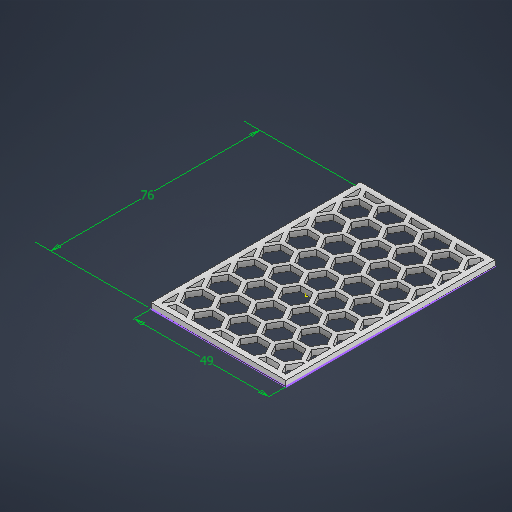
# Autodesk Inventor part: honneypattern
Saved by Autodesk Inventor 2026.1 (Build 301233020, 233B)
## iProperties
Created: 2026-01-08
Part Number: honneypattern
Material: Generic
Document SubType Name: Modeling
Designer: Paweł
Density: 1 g/cm^3
Appearance: Default
Author: Paweł
Autodesk Inventor part; units mm, degrees
ref_plane "YZ Plane" through (0, 0, 0) normal (1, 0, 0) x (0, 1, 0)
ref_plane "XZ Plane" through (0, 0, 0) normal (0, 1, 0) x (-1, 0, 0)
ref_plane "XY Plane" through (0, 0, 0) normal (0, 0, 1) x (1, 0, 0)
sketch "Sketch1" plane through (0, 0, 0) normal (0, 1, 0) x (-1, 0, 0)
  line L0 (23.9507, 32.8498) -> (-25.0493, 32.8498)
  line L1 (-25.0493, 32.8498) -> (-25.0493, -43.1502)
  line L2 (-25.0493, -43.1502) -> (23.9507, -43.1502)
  line L3 (23.9507, -43.1502) -> (23.9507, 32.8498)
  point P0 (0, 0)
  dimension "d0" = 49
  dimension "d1" = 76
  constraints: 8 end point, 2 parallel, 1 horizontal, 1 perpendicular
  measures "d0" distance of L0.start L0.end
  measures "d1" distance of L2.end L0.start
extrude "Extrusion1" add sketch "Sketch1" along normal blind 2
sketch "Sketch2" plane through (0, 2, 0) normal (0, 1, 0) x (1, 0, 0)
  line L0 (2.3094, -38.3498) -> (4.6188, -42.3498)
  line L1 (4.6188, -42.3498) -> (2.3094, -46.3498)
  line L2 (2.3094, -46.3498) -> (-2.3094, -46.3498)
  line L3 (-2.3094, -46.3498) -> (-4.6188, -42.3498)
  line L4 (-4.6188, -42.3498) -> (-2.3094, -38.3498)
  line L5 (-2.3094, -38.3498) -> (2.3094, -38.3498)
  line L6 (-23.9507, -32.8498) -> (25.0493, -32.8498) construction
  line L7 (-23.9507, 43.1502) -> (-23.9507, -32.8498) construction
  line L8 (-23.9507, -32.8498) -> (-23.9507, 0) construction
  line L9 (2.3094, -28.8498) -> (4.6188, -32.8498)
  line L10 (4.6188, -32.8498) -> (2.3094, -36.8498)
  line L11 (2.3094, -36.8498) -> (-2.3094, -36.8498)
  line L12 (-2.3094, -36.8498) -> (-4.6188, -32.8498)
  line L13 (-4.6188, -32.8498) -> (-2.3094, -28.8498)
  line L14 (-2.3094, -28.8498) -> (2.3094, -28.8498)
  line L15 (2.3094, -19.3498) -> (4.6188, -23.3498)
  line L16 (4.6188, -23.3498) -> (2.3094, -27.3498)
  line L17 (2.3094, -27.3498) -> (-2.3094, -27.3498)
  line L18 (-2.3094, -27.3498) -> (-4.6188, -23.3498)
  line L19 (-4.6188, -23.3498) -> (-2.3094, -19.3498)
  line L20 (-2.3094, -19.3498) -> (2.3094, -19.3498)
  line L21 (2.3094, -9.8498) -> (4.6188, -13.8498)
  line L22 (4.6188, -13.8498) -> (2.3094, -17.8498)
  line L23 (2.3094, -17.8498) -> (-2.3094, -17.8498)
  line L24 (-2.3094, -17.8498) -> (-4.6188, -13.8498)
  line L25 (-4.6188, -13.8498) -> (-2.3094, -9.8498)
  line L26 (-2.3094, -9.8498) -> (2.3094, -9.8498)
  line L27 (2.3094, -0.3498) -> (4.6188, -4.3498)
  line L28 (4.6188, -4.3498) -> (2.3094, -8.3498)
  line L29 (2.3094, -8.3498) -> (-2.3094, -8.3498)
  line L30 (-2.3094, -8.3498) -> (-4.6188, -4.3498)
  line L31 (-4.6188, -4.3498) -> (-2.3094, -0.3498)
  line L32 (-2.3094, -0.3498) -> (2.3094, -0.3498)
  line L33 (2.3094, 9.1502) -> (4.6188, 5.1502)
  line L34 (4.6188, 5.1502) -> (2.3094, 1.1502)
  line L35 (2.3094, 1.1502) -> (-2.3094, 1.1502)
  line L36 (-2.3094, 1.1502) -> (-4.6188, 5.1502)
  line L37 (-4.6188, 5.1502) -> (-2.3094, 9.1502)
  line L38 (-2.3094, 9.1502) -> (2.3094, 9.1502)
  line L39 (2.3094, 18.6502) -> (4.6188, 14.6502)
  line L40 (4.6188, 14.6502) -> (2.3094, 10.6502)
  line L41 (2.3094, 10.6502) -> (-2.3094, 10.6502)
  line L42 (-2.3094, 10.6502) -> (-4.6188, 14.6502)
  line L43 (-4.6188, 14.6502) -> (-2.3094, 18.6502)
  line L44 (-2.3094, 18.6502) -> (2.3094, 18.6502)
  line L45 (2.3094, 28.1502) -> (4.6188, 24.1502)
  line L46 (4.6188, 24.1502) -> (2.3094, 20.1502)
  line L47 (2.3094, 20.1502) -> (-2.3094, 20.1502)
  line L48 (-2.3094, 20.1502) -> (-4.6188, 24.1502)
  line L49 (-4.6188, 24.1502) -> (-2.3094, 28.1502)
  line L50 (-2.3094, 28.1502) -> (2.3094, 28.1502)
  line L51 (2.3094, 37.6502) -> (4.6188, 33.6502)
  line L52 (4.6188, 33.6502) -> (2.3094, 29.6502)
  line L53 (2.3094, 29.6502) -> (-2.3094, 29.6502)
  line L54 (-2.3094, 29.6502) -> (-4.6188, 33.6502)
  line L55 (-4.6188, 33.6502) -> (-2.3094, 37.6502)
  line L56 (-2.3094, 37.6502) -> (2.3094, 37.6502)
  line L57 (2.3094, 47.1502) -> (4.6188, 43.1502)
  line L58 (4.6188, 43.1502) -> (2.3094, 39.1502)
  line L59 (2.3094, 39.1502) -> (-2.3094, 39.1502)
  line L60 (-2.3094, 39.1502) -> (-4.6188, 43.1502)
  line L61 (-4.6188, 43.1502) -> (-2.3094, 47.1502)
  line L62 (-2.3094, 47.1502) -> (2.3094, 47.1502)
  line L63 (0, -42.3498) -> (-3.4641, -40.3498) construction
  line L64 (-10.5366, -14.5998) -> (-5.9178, -14.5998)
  line L65 (-5.9178, -13.0998) -> (-10.5366, -13.0998)
  line L66 (-10.5366, -13.0998) -> (-12.846, -9.0998)
  line L67 (-3.6084, -9.0998) -> (-5.9178, -13.0998)
  line L68 (-5.9178, -5.0998) -> (-3.6084, -9.0998)
  line L69 (-10.5366, -5.0998) -> (-5.9178, -5.0998)
  line L70 (-12.846, -9.0998) -> (-10.5366, -5.0998)
  line L71 (-5.9178, -3.5998) -> (-10.5366, -3.5998)
  line L72 (-5.9178, -24.0998) -> (-3.6084, -28.0998)
  line L73 (-12.846, -28.0998) -> (-10.5366, -24.0998)
  line L74 (-5.9178, -14.5998) -> (-3.6084, -18.5998)
  line L75 (-12.846, -18.5998) -> (-10.5366, -14.5998)
  line L76 (-3.6084, -18.5998) -> (-5.9178, -22.5998)
  line L77 (-10.5366, -22.5998) -> (-12.846, -18.5998)
  line L78 (-5.9178, -22.5998) -> (-10.5366, -22.5998)
  line L79 (-10.5366, -24.0998) -> (-5.9178, -24.0998)
  line L80 (-10.5366, -3.5998) -> (-12.846, 0.4002)
  line L81 (-3.6084, 0.4002) -> (-5.9178, -3.5998)
  line L82 (-12.846, 0.4002) -> (-10.5366, 4.4002)
  line L83 (-5.9178, 4.4002) -> (-3.6084, 0.4002)
  line L84 (-10.5366, 4.4002) -> (-5.9178, 4.4002)
  line L85 (-5.9178, 5.9002) -> (-10.5366, 5.9002)
  line L86 (-10.5366, 5.9002) -> (-12.846, 9.9002)
  line L87 (-3.6084, 9.9002) -> (-5.9178, 5.9002)
  line L88 (-12.846, 9.9002) -> (-10.5366, 13.9002)
  line L89 (-5.9178, 13.9002) -> (-3.6084, 9.9002)
  line L90 (-10.5366, 13.9002) -> (-5.9178, 13.9002)
  line L91 (-5.9178, 15.4002) -> (-10.5366, 15.4002)
  line L92 (-10.5366, 15.4002) -> (-12.846, 19.4002)
  line L93 (-3.6084, 19.4002) -> (-5.9178, 15.4002)
  line L94 (-5.9178, -33.5998) -> (-3.6084, -37.5998)
  line L95 (-3.6084, -37.5998) -> (-5.9178, -41.5998)
  line L96 (-5.9178, -41.5998) -> (-10.5366, -41.5998)
  line L97 (-10.5366, -41.5998) -> (-12.846, -37.5998)
  line L98 (-12.846, -37.5998) -> (-10.5366, -33.5998)
  line L99 (-10.5366, -33.5998) -> (-5.9178, -33.5998)
  line L100 (-3.6084, -28.0998) -> (-5.9178, -32.0998)
  line L101 (-5.9178, -32.0998) -> (-10.5366, -32.0998)
  line L102 (-10.5366, -32.0998) -> (-12.846, -28.0998)
  line L103 (-8.2272, -37.5998) -> (-11.6913, -35.5998) construction
  line L104 (-12.846, 19.4002) -> (-10.5366, 23.4002)
  line L105 (-5.9178, 23.4002) -> (-3.6084, 19.4002)
  line L106 (-10.5366, 23.4002) -> (-5.9178, 23.4002)
  line L107 (-5.9178, 24.9002) -> (-10.5366, 24.9002)
  line L108 (-10.5366, 24.9002) -> (-12.846, 28.9002)
  line L109 (-3.6084, 28.9002) -> (-5.9178, 24.9002)
  line L110 (-12.846, 28.9002) -> (-10.5366, 32.9002)
  line L111 (-5.9178, 32.9002) -> (-3.6084, 28.9002)
  line L112 (-5.9178, 34.4002) -> (-10.5366, 34.4002)
  line L113 (-3.6084, 38.4002) -> (-5.9178, 34.4002)
  line L114 (-10.5366, 34.4002) -> (-12.846, 38.4002)
  line L115 (-5.9178, 42.4002) -> (-3.6084, 38.4002)
  line L116 (-10.5366, 42.4002) -> (-5.9178, 42.4002)
  line L117 (-12.846, 38.4002) -> (-10.5366, 42.4002)
  line L118 (-10.5366, 32.9002) -> (-5.9178, 32.9002)
  line L119 (-10.5366, 43.9002) -> (-12.846, 47.9002)
  line L120 (-3.6084, 47.9002) -> (-5.9178, 43.9002)
  line L121 (-12.846, 47.9002) -> (-10.5366, 51.9002)
  line L122 (-10.5366, 51.9002) -> (-5.9178, 51.9002)
  line L123 (-5.9178, 51.9002) -> (-3.6084, 47.9002)
  line L124 (-5.9178, 43.9002) -> (-10.5366, 43.9002)
  line L125 (-18.7639, -9.8498) -> (-14.1451, -9.8498)
  line L126 (-14.1451, -8.3498) -> (-18.7639, -8.3498)
  line L127 (-18.7639, -8.3498) -> (-21.0733, -4.3498)
  line L128 (-11.8357, -4.3498) -> (-14.1451, -8.3498)
  line L129 (-14.1451, -0.3498) -> (-11.8357, -4.3498)
  line L130 (-18.7639, -0.3498) -> (-14.1451, -0.3498)
  line L131 (-21.0733, -4.3498) -> (-18.7639, -0.3498)
  line L132 (-14.1451, 1.1502) -> (-18.7639, 1.1502)
  line L133 (-14.1451, -19.3498) -> (-11.8357, -23.3498)
  line L134 (-21.0733, -23.3498) -> (-18.7639, -19.3498)
  line L135 (-14.1451, -9.8498) -> (-11.8357, -13.8498)
  line L136 (-21.0733, -13.8498) -> (-18.7639, -9.8498)
  line L137 (-11.8357, -13.8498) -> (-14.1451, -17.8498)
  line L138 (-18.7639, -17.8498) -> (-21.0733, -13.8498)
  line L139 (-14.1451, -17.8498) -> (-18.7639, -17.8498)
  line L140 (-18.7639, -19.3498) -> (-14.1451, -19.3498)
  line L141 (-18.7639, 1.1502) -> (-21.0733, 5.1502)
  line L142 (-11.8357, 5.1502) -> (-14.1451, 1.1502)
  line L143 (-21.0733, 5.1502) -> (-18.7639, 9.1502)
  line L144 (-14.1451, 9.1502) -> (-11.8357, 5.1502)
  line L145 (-18.7639, 9.1502) -> (-14.1451, 9.1502)
  line L146 (-14.1451, 10.6502) -> (-18.7639, 10.6502)
  line L147 (-18.7639, 10.6502) -> (-21.0733, 14.6502)
  line L148 (-11.8357, 14.6502) -> (-14.1451, 10.6502)
  line L149 (-21.0733, 14.6502) -> (-18.7639, 18.6502)
  line L150 (-14.1451, 18.6502) -> (-11.8357, 14.6502)
  line L151 (-18.7639, 18.6502) -> (-14.1451, 18.6502)
  line L152 (-14.1451, 20.1502) -> (-18.7639, 20.1502)
  line L153 (-18.7639, 20.1502) -> (-21.0733, 24.1502)
  line L154 (-11.8357, 24.1502) -> (-14.1451, 20.1502)
  line L155 (-14.1451, -28.8498) -> (-11.8357, -32.8498)
  line L156 (-11.8357, -32.8498) -> (-14.1451, -36.8498)
  line L157 (-14.1451, -36.8498) -> (-18.7639, -36.8498)
  line L158 (-18.7639, -36.8498) -> (-21.0733, -32.8498)
  line L159 (-21.0733, -32.8498) -> (-18.7639, -28.8498)
  line L160 (-18.7639, -28.8498) -> (-14.1451, -28.8498)
  line L161 (-11.8357, -23.3498) -> (-14.1451, -27.3498)
  line L162 (-14.1451, -27.3498) -> (-18.7639, -27.3498)
  line L163 (-18.7639, -27.3498) -> (-21.0733, -23.3498)
  line L164 (-16.4545, -32.8498) -> (-19.9186, -30.8498) construction
  line L165 (-21.0733, 24.1502) -> (-18.7639, 28.1502)
  line L166 (-14.1451, 28.1502) -> (-11.8357, 24.1502)
  line L167 (-18.7639, 28.1502) -> (-14.1451, 28.1502)
  line L168 (-14.1451, 29.6502) -> (-18.7639, 29.6502)
  line L169 (-18.7639, 29.6502) -> (-21.0733, 33.6502)
  line L170 (-11.8357, 33.6502) -> (-14.1451, 29.6502)
  line L171 (-21.0733, 33.6502) -> (-18.7639, 37.6502)
  line L172 (-14.1451, 37.6502) -> (-11.8357, 33.6502)
  line L173 (-14.1451, 39.1502) -> (-18.7639, 39.1502)
  line L174 (-11.8357, 43.1502) -> (-14.1451, 39.1502)
  line L175 (-18.7639, 39.1502) -> (-21.0733, 43.1502)
  line L176 (-14.1451, 47.1502) -> (-11.8357, 43.1502)
  line L177 (-18.7639, 47.1502) -> (-14.1451, 47.1502)
  line L178 (-21.0733, 43.1502) -> (-18.7639, 47.1502)
  line L179 (-18.7639, 37.6502) -> (-14.1451, 37.6502)
  line L180 (-18.7639, 48.6502) -> (-21.0733, 52.6502)
  line L181 (-11.8357, 52.6502) -> (-14.1451, 48.6502)
  line L182 (-21.0733, 52.6502) -> (-18.7639, 56.6502)
  line L183 (-18.7639, 56.6502) -> (-14.1451, 56.6502)
  line L184 (-14.1451, 56.6502) -> (-11.8357, 52.6502)
  line L185 (-14.1451, 48.6502) -> (-18.7639, 48.6502)
  line L186 (-26.9911, -5.0998) -> (-22.3723, -5.0998)
  line L187 (-22.3723, -3.5998) -> (-26.9911, -3.5998)
  line L188 (-26.9911, -3.5998) -> (-29.3005, 0.4002)
  line L189 (-20.0629, 0.4002) -> (-22.3723, -3.5998)
  line L190 (-22.3723, 4.4002) -> (-20.0629, 0.4002)
  line L191 (-26.9911, 4.4002) -> (-22.3723, 4.4002)
  line L192 (-29.3005, 0.4002) -> (-26.9911, 4.4002)
  line L193 (-22.3723, 5.9002) -> (-26.9911, 5.9002)
  line L194 (-22.3723, -14.5998) -> (-20.0629, -18.5998)
  line L195 (-29.3005, -18.5998) -> (-26.9911, -14.5998)
  line L196 (-22.3723, -5.0998) -> (-20.0629, -9.0998)
  line L197 (-29.3005, -9.0998) -> (-26.9911, -5.0998)
  line L198 (-20.0629, -9.0998) -> (-22.3723, -13.0998)
  line L199 (-26.9911, -13.0998) -> (-29.3005, -9.0998)
  line L200 (-22.3723, -13.0998) -> (-26.9911, -13.0998)
  line L201 (-26.9911, -14.5998) -> (-22.3723, -14.5998)
  line L202 (-26.9911, 5.9002) -> (-29.3005, 9.9002)
  line L203 (-20.0629, 9.9002) -> (-22.3723, 5.9002)
  line L204 (-29.3005, 9.9002) -> (-26.9911, 13.9002)
  line L205 (-22.3723, 13.9002) -> (-20.0629, 9.9002)
  line L206 (-26.9911, 13.9002) -> (-22.3723, 13.9002)
  line L207 (-22.3723, 15.4002) -> (-26.9911, 15.4002)
  line L208 (-26.9911, 15.4002) -> (-29.3005, 19.4002)
  line L209 (-20.0629, 19.4002) -> (-22.3723, 15.4002)
  line L210 (-29.3005, 19.4002) -> (-26.9911, 23.4002)
  line L211 (-22.3723, 23.4002) -> (-20.0629, 19.4002)
  line L212 (-26.9911, 23.4002) -> (-22.3723, 23.4002)
  line L213 (-22.3723, 24.9002) -> (-26.9911, 24.9002)
  line L214 (-26.9911, 24.9002) -> (-29.3005, 28.9002)
  line L215 (-20.0629, 28.9002) -> (-22.3723, 24.9002)
  line L216 (-22.3723, -24.0998) -> (-20.0629, -28.0998)
  line L217 (-20.0629, -28.0998) -> (-22.3723, -32.0998)
  line L218 (-22.3723, -32.0998) -> (-26.9911, -32.0998)
  line L219 (-26.9911, -32.0998) -> (-29.3005, -28.0998)
  line L220 (-29.3005, -28.0998) -> (-26.9911, -24.0998)
  line L221 (-26.9911, -24.0998) -> (-22.3723, -24.0998)
  line L222 (-20.0629, -18.5998) -> (-22.3723, -22.5998)
  line L223 (-22.3723, -22.5998) -> (-26.9911, -22.5998)
  line L224 (-26.9911, -22.5998) -> (-29.3005, -18.5998)
  line L225 (-24.6817, -28.0998) -> (-28.1458, -26.0998) construction
  line L226 (-29.3005, 28.9002) -> (-26.9911, 32.9002)
  line L227 (-22.3723, 32.9002) -> (-20.0629, 28.9002)
  line L228 (-26.9911, 32.9002) -> (-22.3723, 32.9002)
  line L229 (-22.3723, 34.4002) -> (-26.9911, 34.4002)
  line L230 (-26.9911, 34.4002) -> (-29.3005, 38.4002)
  line L231 (-20.0629, 38.4002) -> (-22.3723, 34.4002)
  line L232 (-29.3005, 38.4002) -> (-26.9911, 42.4002)
  line L233 (-22.3723, 42.4002) -> (-20.0629, 38.4002)
  line L234 (-22.3723, 43.9002) -> (-26.9911, 43.9002)
  line L235 (-20.0629, 47.9002) -> (-22.3723, 43.9002)
  line L236 (-26.9911, 43.9002) -> (-29.3005, 47.9002)
  line L237 (-22.3723, 51.9002) -> (-20.0629, 47.9002)
  line L238 (-26.9911, 51.9002) -> (-22.3723, 51.9002)
  line L239 (-29.3005, 47.9002) -> (-26.9911, 51.9002)
  line L240 (-26.9911, 42.4002) -> (-22.3723, 42.4002)
  line L241 (-26.9911, 53.4002) -> (-29.3005, 57.4002)
  line L242 (-20.0629, 57.4002) -> (-22.3723, 53.4002)
  line L243 (-29.3005, 57.4002) -> (-26.9911, 61.4002)
  line L244 (-26.9911, 61.4002) -> (-22.3723, 61.4002)
  line L245 (-22.3723, 61.4002) -> (-20.0629, 57.4002)
  line L246 (-22.3723, 53.4002) -> (-26.9911, 53.4002)
  line L247 (10.5366, -43.0998) -> (12.846, -47.0998)
  line L248 (12.846, -47.0998) -> (10.5366, -51.0998)
  line L249 (10.5366, -51.0998) -> (5.9178, -51.0998)
  line L250 (5.9178, -51.0998) -> (3.6084, -47.0998)
  line L251 (3.6084, -47.0998) -> (5.9178, -43.0998)
  line L252 (8.2272, -47.0998) -> (4.7631, -45.0998) construction
  line L253 (12.846, -37.5998) -> (10.5366, -41.5998)
  line L254 (10.5366, -24.0998) -> (12.846, -28.0998)
  line L255 (12.846, -28.0998) -> (10.5366, -32.0998)
  line L256 (5.9178, -32.0998) -> (3.6084, -28.0998)
  line L257 (3.6084, -28.0998) -> (5.9178, -24.0998)
  line L258 (5.9178, -22.5998) -> (3.6084, -18.5998)
  line L259 (5.9178, -24.0998) -> (10.5366, -24.0998)
  line L260 (12.846, -9.0998) -> (10.5366, -13.0998)
  line L261 (10.5366, -13.0998) -> (5.9178, -13.0998)
  line L262 (5.9178, -14.5998) -> (10.5366, -14.5998)
  line L263 (10.5366, -14.5998) -> (12.846, -18.5998)
  line L264 (12.846, -18.5998) -> (10.5366, -22.5998)
  line L265 (10.5366, -22.5998) -> (5.9178, -22.5998)
  line L266 (3.6084, -18.5998) -> (5.9178, -14.5998)
  line L267 (5.9178, -13.0998) -> (3.6084, -9.0998)
  line L268 (5.9178, -3.5998) -> (3.6084, 0.4002)
  line L269 (3.6084, -9.0998) -> (5.9178, -5.0998)
  line L270 (5.9178, -5.0998) -> (10.5366, -5.0998)
  line L271 (10.5366, -3.5998) -> (5.9178, -3.5998)
  line L272 (10.5366, -5.0998) -> (12.846, -9.0998)
  line L273 (12.846, 0.4002) -> (10.5366, -3.5998)
  line L274 (10.5366, 4.4002) -> (12.846, 0.4002)
  line L275 (3.6084, 0.4002) -> (5.9178, 4.4002)
  line L276 (5.9178, 4.4002) -> (10.5366, 4.4002)
  line L277 (5.9178, 5.9002) -> (3.6084, 9.9002)
  line L278 (3.6084, 9.9002) -> (5.9178, 13.9002)
  line L279 (12.846, 9.9002) -> (10.5366, 5.9002)
  line L280 (5.9178, 13.9002) -> (10.5366, 13.9002)
  line L281 (10.5366, 15.4002) -> (5.9178, 15.4002)
  line L282 (10.5366, 13.9002) -> (12.846, 9.9002)
  line L283 (12.846, 19.4002) -> (10.5366, 15.4002)
  line L284 (10.5366, 5.9002) -> (5.9178, 5.9002)
  line L285 (5.9178, 15.4002) -> (3.6084, 19.4002)
  line L286 (3.6084, 19.4002) -> (5.9178, 23.4002)
  line L287 (3.6084, 28.9002) -> (5.9178, 32.9002)
  line L288 (5.9178, 24.9002) -> (3.6084, 28.9002)
  line L289 (10.5366, 32.9002) -> (12.846, 28.9002)
  line L290 (10.5366, 24.9002) -> (5.9178, 24.9002)
  line L291 (5.9178, 23.4002) -> (10.5366, 23.4002)
  line L292 (12.846, 28.9002) -> (10.5366, 24.9002)
  line L293 (10.5366, 23.4002) -> (12.846, 19.4002)
  line L294 (5.9178, 32.9002) -> (10.5366, 32.9002)
  line L295 (3.6084, 38.4002) -> (5.9178, 42.4002)
  line L296 (5.9178, 42.4002) -> (10.5366, 42.4002)
  line L297 (10.5366, 34.4002) -> (5.9178, 34.4002)
  line L298 (10.5366, 42.4002) -> (12.846, 38.4002)
  line L299 (12.846, 38.4002) -> (10.5366, 34.4002)
  line L300 (5.9178, 34.4002) -> (3.6084, 38.4002)
  line L301 (10.5366, -41.5998) -> (5.9178, -41.5998)
  line L302 (5.9178, -43.0998) -> (10.5366, -43.0998)
  line L303 (10.5366, -33.5998) -> (12.846, -37.5998)
  line L304 (5.9178, -41.5998) -> (3.6084, -37.5998)
  line L305 (5.9178, -33.5998) -> (10.5366, -33.5998)
  line L306 (10.5366, -32.0998) -> (5.9178, -32.0998)
  line L307 (3.6084, -37.5998) -> (5.9178, -33.5998)
  line L308 (18.7639, -47.8498) -> (21.0733, -51.8498)
  line L309 (21.0733, -51.8498) -> (18.7639, -55.8498)
  line L310 (18.7639, -55.8498) -> (14.1451, -55.8498)
  line L311 (14.1451, -55.8498) -> (11.8357, -51.8498)
  line L312 (11.8357, -51.8498) -> (14.1451, -47.8498)
  line L313 (16.4545, -51.8498) -> (12.9904, -49.8498) construction
  line L314 (21.0733, -42.3498) -> (18.7639, -46.3498)
  line L315 (18.7639, -28.8498) -> (21.0733, -32.8498)
  line L316 (21.0733, -32.8498) -> (18.7639, -36.8498)
  line L317 (14.1451, -36.8498) -> (11.8357, -32.8498)
  line L318 (11.8357, -32.8498) -> (14.1451, -28.8498)
  line L319 (14.1451, -27.3498) -> (11.8357, -23.3498)
  line L320 (14.1451, -28.8498) -> (18.7639, -28.8498)
  line L321 (21.0733, -13.8498) -> (18.7639, -17.8498)
  line L322 (18.7639, -17.8498) -> (14.1451, -17.8498)
  line L323 (14.1451, -19.3498) -> (18.7639, -19.3498)
  line L324 (18.7639, -19.3498) -> (21.0733, -23.3498)
  line L325 (21.0733, -23.3498) -> (18.7639, -27.3498)
  line L326 (18.7639, -27.3498) -> (14.1451, -27.3498)
  line L327 (11.8357, -23.3498) -> (14.1451, -19.3498)
  line L328 (14.1451, -17.8498) -> (11.8357, -13.8498)
  line L329 (14.1451, -8.3498) -> (11.8357, -4.3498)
  line L330 (11.8357, -13.8498) -> (14.1451, -9.8498)
  line L331 (14.1451, -9.8498) -> (18.7639, -9.8498)
  line L332 (18.7639, -8.3498) -> (14.1451, -8.3498)
  line L333 (18.7639, -9.8498) -> (21.0733, -13.8498)
  line L334 (21.0733, -4.3498) -> (18.7639, -8.3498)
  line L335 (18.7639, -0.3498) -> (21.0733, -4.3498)
  line L336 (11.8357, -4.3498) -> (14.1451, -0.3498)
  line L337 (14.1451, -0.3498) -> (18.7639, -0.3498)
  line L338 (14.1451, 1.1502) -> (11.8357, 5.1502)
  line L339 (11.8357, 5.1502) -> (14.1451, 9.1502)
  line L340 (21.0733, 5.1502) -> (18.7639, 1.1502)
  line L341 (14.1451, 9.1502) -> (18.7639, 9.1502)
  line L342 (18.7639, 10.6502) -> (14.1451, 10.6502)
  line L343 (18.7639, 9.1502) -> (21.0733, 5.1502)
  line L344 (21.0733, 14.6502) -> (18.7639, 10.6502)
  line L345 (18.7639, 1.1502) -> (14.1451, 1.1502)
  line L346 (14.1451, 10.6502) -> (11.8357, 14.6502)
  line L347 (11.8357, 14.6502) -> (14.1451, 18.6502)
  line L348 (11.8357, 24.1502) -> (14.1451, 28.1502)
  line L349 (14.1451, 20.1502) -> (11.8357, 24.1502)
  line L350 (18.7639, 28.1502) -> (21.0733, 24.1502)
  line L351 (18.7639, 20.1502) -> (14.1451, 20.1502)
  line L352 (14.1451, 18.6502) -> (18.7639, 18.6502)
  line L353 (21.0733, 24.1502) -> (18.7639, 20.1502)
  line L354 (18.7639, 18.6502) -> (21.0733, 14.6502)
  line L355 (14.1451, 28.1502) -> (18.7639, 28.1502)
  line L356 (11.8357, 33.6502) -> (14.1451, 37.6502)
  line L357 (14.1451, 37.6502) -> (18.7639, 37.6502)
  line L358 (18.7639, 29.6502) -> (14.1451, 29.6502)
  line L359 (18.7639, 37.6502) -> (21.0733, 33.6502)
  line L360 (21.0733, 33.6502) -> (18.7639, 29.6502)
  line L361 (14.1451, 29.6502) -> (11.8357, 33.6502)
  line L362 (18.7639, -46.3498) -> (14.1451, -46.3498)
  line L363 (14.1451, -47.8498) -> (18.7639, -47.8498)
  line L364 (18.7639, -38.3498) -> (21.0733, -42.3498)
  line L365 (14.1451, -46.3498) -> (11.8357, -42.3498)
  line L366 (14.1451, -38.3498) -> (18.7639, -38.3498)
  line L367 (18.7639, -36.8498) -> (14.1451, -36.8498)
  line L368 (11.8357, -42.3498) -> (14.1451, -38.3498)
  line L369 (26.9911, -52.5998) -> (29.3005, -56.5998)
  line L370 (29.3005, -56.5998) -> (26.9911, -60.5998)
  line L371 (26.9911, -60.5998) -> (22.3723, -60.5998)
  line L372 (22.3723, -60.5998) -> (20.0629, -56.5998)
  line L373 (20.0629, -56.5998) -> (22.3723, -52.5998)
  line L374 (24.6817, -56.5998) -> (21.2176, -54.5998) construction
  line L375 (29.3005, -47.0998) -> (26.9911, -51.0998)
  line L376 (26.9911, -33.5998) -> (29.3005, -37.5998)
  line L377 (29.3005, -37.5998) -> (26.9911, -41.5998)
  line L378 (22.3723, -41.5998) -> (20.0629, -37.5998)
  line L379 (20.0629, -37.5998) -> (22.3723, -33.5998)
  line L380 (22.3723, -32.0998) -> (20.0629, -28.0998)
  line L381 (22.3723, -33.5998) -> (26.9911, -33.5998)
  line L382 (29.3005, -18.5998) -> (26.9911, -22.5998)
  line L383 (26.9911, -22.5998) -> (22.3723, -22.5998)
  line L384 (22.3723, -24.0998) -> (26.9911, -24.0998)
  line L385 (26.9911, -24.0998) -> (29.3005, -28.0998)
  line L386 (29.3005, -28.0998) -> (26.9911, -32.0998)
  line L387 (26.9911, -32.0998) -> (22.3723, -32.0998)
  line L388 (20.0629, -28.0998) -> (22.3723, -24.0998)
  line L389 (22.3723, -22.5998) -> (20.0629, -18.5998)
  line L390 (22.3723, -13.0998) -> (20.0629, -9.0998)
  line L391 (20.0629, -18.5998) -> (22.3723, -14.5998)
  line L392 (22.3723, -14.5998) -> (26.9911, -14.5998)
  line L393 (26.9911, -13.0998) -> (22.3723, -13.0998)
  line L394 (26.9911, -14.5998) -> (29.3005, -18.5998)
  line L395 (29.3005, -9.0998) -> (26.9911, -13.0998)
  line L396 (26.9911, -5.0998) -> (29.3005, -9.0998)
  line L397 (20.0629, -9.0998) -> (22.3723, -5.0998)
  line L398 (22.3723, -5.0998) -> (26.9911, -5.0998)
  line L399 (22.3723, -3.5998) -> (20.0629, 0.4002)
  line L400 (20.0629, 0.4002) -> (22.3723, 4.4002)
  line L401 (29.3005, 0.4002) -> (26.9911, -3.5998)
  line L402 (22.3723, 4.4002) -> (26.9911, 4.4002)
  line L403 (26.9911, 5.9002) -> (22.3723, 5.9002)
  line L404 (26.9911, 4.4002) -> (29.3005, 0.4002)
  line L405 (29.3005, 9.9002) -> (26.9911, 5.9002)
  line L406 (26.9911, -3.5998) -> (22.3723, -3.5998)
  line L407 (22.3723, 5.9002) -> (20.0629, 9.9002)
  line L408 (20.0629, 9.9002) -> (22.3723, 13.9002)
  line L409 (20.0629, 19.4002) -> (22.3723, 23.4002)
  line L410 (22.3723, 15.4002) -> (20.0629, 19.4002)
  line L411 (26.9911, 23.4002) -> (29.3005, 19.4002)
  line L412 (26.9911, 15.4002) -> (22.3723, 15.4002)
  line L413 (22.3723, 13.9002) -> (26.9911, 13.9002)
  line L414 (29.3005, 19.4002) -> (26.9911, 15.4002)
  line L415 (26.9911, 13.9002) -> (29.3005, 9.9002)
  line L416 (22.3723, 23.4002) -> (26.9911, 23.4002)
  line L417 (20.0629, 28.9002) -> (22.3723, 32.9002)
  line L418 (22.3723, 32.9002) -> (26.9911, 32.9002)
  line L419 (26.9911, 24.9002) -> (22.3723, 24.9002)
  line L420 (26.9911, 32.9002) -> (29.3005, 28.9002)
  line L421 (29.3005, 28.9002) -> (26.9911, 24.9002)
  line L422 (22.3723, 24.9002) -> (20.0629, 28.9002)
  line L423 (26.9911, -51.0998) -> (22.3723, -51.0998)
  line L424 (22.3723, -52.5998) -> (26.9911, -52.5998)
  line L425 (26.9911, -43.0998) -> (29.3005, -47.0998)
  line L426 (22.3723, -51.0998) -> (20.0629, -47.0998)
  line L427 (22.3723, -43.0998) -> (26.9911, -43.0998)
  line L428 (26.9911, -41.5998) -> (22.3723, -41.5998)
  line L429 (20.0629, -47.0998) -> (22.3723, -43.0998)
  line L430 (35.2184, -57.3498) -> (37.5278, -61.3498)
  line L431 (37.5278, -61.3498) -> (35.2184, -65.3498)
  line L432 (35.2184, -65.3498) -> (30.5996, -65.3498)
  line L433 (30.5996, -65.3498) -> (28.2902, -61.3498)
  line L434 (28.2902, -61.3498) -> (30.5996, -57.3498)
  line L435 (32.909, -61.3498) -> (29.4449, -59.3498) construction
  line L436 (37.5278, -51.8498) -> (35.2184, -55.8498)
  line L437 (35.2184, -38.3498) -> (37.5278, -42.3498)
  line L438 (37.5278, -42.3498) -> (35.2184, -46.3498)
  line L439 (30.5996, -46.3498) -> (28.2902, -42.3498)
  line L440 (28.2902, -42.3498) -> (30.5996, -38.3498)
  line L441 (30.5996, -36.8498) -> (28.2902, -32.8498)
  line L442 (30.5996, -38.3498) -> (35.2184, -38.3498)
  line L443 (37.5278, -23.3498) -> (35.2184, -27.3498)
  line L444 (35.2184, -27.3498) -> (30.5996, -27.3498)
  line L445 (30.5996, -28.8498) -> (35.2184, -28.8498)
  line L446 (35.2184, -28.8498) -> (37.5278, -32.8498)
  line L447 (37.5278, -32.8498) -> (35.2184, -36.8498)
  line L448 (35.2184, -36.8498) -> (30.5996, -36.8498)
  line L449 (28.2902, -32.8498) -> (30.5996, -28.8498)
  line L450 (30.5996, -27.3498) -> (28.2902, -23.3498)
  line L451 (30.5996, -17.8498) -> (28.2902, -13.8498)
  line L452 (28.2902, -23.3498) -> (30.5996, -19.3498)
  line L453 (30.5996, -19.3498) -> (35.2184, -19.3498)
  line L454 (35.2184, -17.8498) -> (30.5996, -17.8498)
  line L455 (35.2184, -19.3498) -> (37.5278, -23.3498)
  line L456 (37.5278, -13.8498) -> (35.2184, -17.8498)
  line L457 (35.2184, -9.8498) -> (37.5278, -13.8498)
  line L458 (28.2902, -13.8498) -> (30.5996, -9.8498)
  line L459 (30.5996, -9.8498) -> (35.2184, -9.8498)
  line L460 (30.5996, -8.3498) -> (28.2902, -4.3498)
  line L461 (28.2902, -4.3498) -> (30.5996, -0.3498)
  line L462 (37.5278, -4.3498) -> (35.2184, -8.3498)
  line L463 (30.5996, -0.3498) -> (35.2184, -0.3498)
  line L464 (35.2184, 1.1502) -> (30.5996, 1.1502)
  line L465 (35.2184, -0.3498) -> (37.5278, -4.3498)
  line L466 (37.5278, 5.1502) -> (35.2184, 1.1502)
  line L467 (35.2184, -8.3498) -> (30.5996, -8.3498)
  line L468 (30.5996, 1.1502) -> (28.2902, 5.1502)
  line L469 (28.2902, 5.1502) -> (30.5996, 9.1502)
  line L470 (28.2902, 14.6502) -> (30.5996, 18.6502)
  line L471 (30.5996, 10.6502) -> (28.2902, 14.6502)
  line L472 (35.2184, 18.6502) -> (37.5278, 14.6502)
  line L473 (35.2184, 10.6502) -> (30.5996, 10.6502)
  line L474 (30.5996, 9.1502) -> (35.2184, 9.1502)
  line L475 (37.5278, 14.6502) -> (35.2184, 10.6502)
  line L476 (35.2184, 9.1502) -> (37.5278, 5.1502)
  line L477 (30.5996, 18.6502) -> (35.2184, 18.6502)
  line L478 (28.2902, 24.1502) -> (30.5996, 28.1502)
  line L479 (30.5996, 28.1502) -> (35.2184, 28.1502)
  line L480 (35.2184, 20.1502) -> (30.5996, 20.1502)
  line L481 (35.2184, 28.1502) -> (37.5278, 24.1502)
  line L482 (37.5278, 24.1502) -> (35.2184, 20.1502)
  line L483 (30.5996, 20.1502) -> (28.2902, 24.1502)
  line L484 (35.2184, -55.8498) -> (30.5996, -55.8498)
  line L485 (30.5996, -57.3498) -> (35.2184, -57.3498)
  line L486 (35.2184, -47.8498) -> (37.5278, -51.8498)
  line L487 (30.5996, -55.8498) -> (28.2902, -51.8498)
  line L488 (30.5996, -47.8498) -> (35.2184, -47.8498)
  line L489 (35.2184, -46.3498) -> (30.5996, -46.3498)
  line L490 (28.2902, -51.8498) -> (30.5996, -47.8498)
  line L491 (18.7639, 47.1502) -> (21.0733, 43.1502)
  line L492 (14.1451, 47.1502) -> (18.7639, 47.1502)
  line L493 (11.8357, 43.1502) -> (14.1451, 47.1502)
  line L494 (14.1451, 39.1502) -> (11.8357, 43.1502)
  line L495 (18.7639, 39.1502) -> (14.1451, 39.1502)
  line L496 (21.0733, 43.1502) -> (18.7639, 39.1502)
  line L497 (22.3723, 34.4002) -> (20.0629, 38.4002)
  line L498 (26.9911, 34.4002) -> (22.3723, 34.4002)
  line L499 (29.3005, 38.4002) -> (26.9911, 34.4002)
  line L500 (26.9911, 42.4002) -> (29.3005, 38.4002)
  line L501 (22.3723, 42.4002) -> (26.9911, 42.4002)
  line L502 (20.0629, 38.4002) -> (22.3723, 42.4002)
  line L503 (-23.9507, -23.3498) -> (-23.9507, 9.5) construction
  point P0 (0, 0)
  point P1 (0, -38.3498)
  point P2 (0, -32.8498)
  point P3 (0, -28.8498)
  point P4 (0, -23.3498)
  point P5 (0, -19.3498)
  point P6 (0, -13.8498)
  point P7 (0, -9.8498)
  point P8 (0, -4.3498)
  point P9 (0, -0.3498)
  point P10 (0, 5.1502)
  point P11 (0, 9.1502)
  point P12 (0, 14.6502)
  point P13 (0, 18.6502)
  point P14 (0, 24.1502)
  point P15 (0, 28.1502)
  point P16 (0, 33.6502)
  point P17 (0, 37.6502)
  point P18 (0, 43.1502)
  point P19 (0, 47.1502)
  point P20 (-8.2272, -14.5998)
  point P21 (-8.2272, -9.0998)
  point P22 (-8.2272, -5.0998)
  point P23 (-8.2272, 4.75)
  point P24 (-8.2272, -28.0998)
  point P25 (-8.2272, -18.5998)
  point P26 (-8.2272, -24.0998)
  point P27 (-8.2272, 0.4002)
  point P28 (-8.2272, 4.4002)
  point P29 (-8.2272, 9.9002)
  point P30 (-8.2272, 13.9002)
  point P31 (-8.2272, -33.5998)
  point P32 (-8.2272, 19.4002)
  point P33 (-8.2272, 23.4002)
  point P34 (-8.2272, 28.9002)
  point P35 (-8.2272, 32.9002)
  point P36 (-8.2272, 38.4002)
  point P37 (-8.2272, 42.4002)
  point P38 (-8.2272, 47.9002)
  point P39 (-8.2272, 51.9002)
  point P40 (-16.4545, -9.8498)
  point P41 (-16.4545, -4.3498)
  point P42 (-16.4545, -0.3498)
  point P43 (-16.4545, 9.5)
  point P44 (-16.4545, -23.3498)
  point P45 (-16.4545, -13.8498)
  point P46 (-16.4545, -19.3498)
  point P47 (-16.4545, 5.1502)
  point P48 (-16.4545, 9.1502)
  point P49 (-16.4545, 14.6502)
  point P50 (-16.4545, 18.6502)
  point P51 (-16.4545, -28.8498)
  point P52 (-16.4545, 24.1502)
  point P53 (-16.4545, 28.1502)
  point P54 (-16.4545, 33.6502)
  point P55 (-16.4545, 37.6502)
  point P56 (-16.4545, 43.1502)
  point P57 (-16.4545, 47.1502)
  point P58 (-16.4545, 52.6502)
  point P59 (-16.4545, 56.6502)
  point P60 (-24.6817, -5.0998)
  point P61 (-24.6817, 0.4002)
  point P62 (-24.6817, 4.4002)
  point P63 (-24.6817, 14.25)
  point P64 (-24.6817, -18.5998)
  point P65 (-24.6817, -9.0998)
  point P66 (-24.6817, -14.5998)
  point P67 (-24.6817, 9.9002)
  point P68 (-24.6817, 13.9002)
  point P69 (-24.6817, 19.4002)
  point P70 (-24.6817, 23.4002)
  point P71 (-24.6817, -24.0998)
  point P72 (-24.6817, 28.9002)
  point P73 (-24.6817, 32.9002)
  point P74 (-24.6817, 38.4002)
  point P75 (-24.6817, 42.4002)
  point P76 (-24.6817, 47.9002)
  point P77 (-24.6817, 51.9002)
  point P78 (-24.6817, 57.4002)
  point P79 (-24.6817, 61.4002)
  point P80 (8.2272, -43.0998)
  point P81 (2.3094, -38.3498)
  point P82 (8.2272, -37.5998)
  point P83 (8.2272, -28.0998)
  point P84 (2.3094, -28.8498)
  point P85 (8.2272, -24.0998)
  point P86 (8.2272, -18.5998)
  point P87 (8.2272, -9.0998)
  point P88 (8.2272, -14.5998)
  point P89 (8.2272, -4.75)
  point P90 (8.2272, 0.4002)
  point P91 (8.2272, -5.0998)
  point P92 (8.2272, 4.4002)
  point P93 (8.2272, 9.9002)
  point P94 (8.2272, 13.9002)
  point P95 (8.2272, 19.4002)
  point P96 (8.2272, 23.4002)
  point P97 (8.2272, 28.9002)
  point P98 (8.2272, 32.9002)
  point P99 (8.2272, 38.4002)
  point P100 (8.2272, 42.4002)
  point P101 (8.2272, -33.5998)
  point P102 (16.4545, -47.8498)
  point P103 (10.5366, -51.0998)
  point P104 (16.4545, -42.3498)
  point P105 (16.4545, -32.8498)
  point P106 (10.5366, -33.5998)
  point P107 (12.846, -37.5998)
  point P108 (10.5366, -32.0998)
  point P109 (16.4545, -28.8498)
  point P110 (16.4545, -23.3498)
  point P111 (16.4545, -13.8498)
  point P112 (16.4545, -19.3498)
  point P113 (12.846, -18.5998)
  point P114 (16.4545, -9.5)
  point P115 (16.4545, -4.3498)
  point P116 (16.4545, -9.8498)
  point P117 (12.846, 0.4002)
  point P118 (16.4545, -0.3498)
  point P119 (16.4545, 5.1502)
  point P120 (16.4545, 9.1502)
  point P121 (16.4545, 14.6502)
  point P122 (12.846, 9.9002)
  point P123 (12.846, 19.4002)
  point P124 (16.4545, 18.6502)
  point P125 (16.4545, 24.1502)
  point P126 (16.4545, 28.1502)
  point P127 (16.4545, 33.6502)
  point P128 (12.846, 28.9002)
  point P129 (16.4545, 37.6502)
  point P130 (16.4545, -38.3498)
  point P131 (24.6817, -52.5998)
  point P132 (21.0733, -51.8498)
  point P133 (24.6817, -47.0998)
  point P134 (24.6817, -37.5998)
  point P135 (21.0733, -42.3498)
  point P136 (21.0733, -32.8498)
  point P137 (24.6817, -33.5998)
  point P138 (24.6817, -28.0998)
  point P139 (24.6817, -18.5998)
  point P140 (24.6817, -24.0998)
  point P141 (21.0733, -13.8498)
  point P142 (24.6817, -14.25)
  point P143 (24.6817, -9.0998)
  point P144 (24.6817, -14.5998)
  point P145 (21.0733, -4.3498)
  point P146 (24.6817, -5.0998)
  point P147 (24.6817, 0.4002)
  point P148 (24.6817, 4.4002)
  point P149 (24.6817, 9.9002)
  point P150 (21.0733, 5.1502)
  point P151 (24.6817, 13.9002)
  point P152 (24.6817, 19.4002)
  point P153 (24.6817, 23.4002)
  point P154 (24.6817, 28.9002)
  point P155 (21.0733, 24.1502)
  point P156 (24.6817, 32.9002)
  point P157 (21.0733, 33.6502)
  point P158 (24.6817, -43.0998)
  point P159 (18.7639, -46.3498)
  point P160 (32.909, -57.3498)
  point P161 (32.909, -51.8498)
  point P162 (32.909, -42.3498)
  point P163 (29.3005, -47.0998)
  point P164 (32.909, -38.3498)
  point P165 (32.909, -32.8498)
  point P166 (32.909, -23.3498)
  point P167 (32.909, -28.8498)
  point P168 (32.909, -19)
  point P169 (32.909, -13.8498)
  point P170 (32.909, -19.3498)
  point P171 (29.3005, -9.0998)
  point P172 (32.909, -9.8498)
  point P173 (32.909, -4.3498)
  point P174 (32.909, -0.3498)
  point P175 (32.909, 5.1502)
  point P176 (29.3005, 9.9002)
  point P177 (32.909, 9.1502)
  point P178 (32.909, 14.6502)
  point P179 (32.909, 18.6502)
  point P180 (32.909, 24.1502)
  point P181 (29.3005, 19.4002)
  point P182 (32.909, 28.1502)
  point P183 (29.3005, 28.9002)
  point P184 (32.909, -47.8498)
  point P185 (26.9911, -51.0998)
  point P186 (16.4545, 47.1502)
  point P187 (24.6817, 42.4002)
  dimension "d4" = 8
  dimension "d5" = 9.5
  dimension "d8" = 9.5
  dimension "d15" = 9.5
  dimension "d22" = 9.5
  dimension "d29" = 9.5
  constraints: 1004 end point, 2 collinear, 2 midpoint, 2 vertical, 2 vertical alignment, 1 horizontal, 1 horizontal alignment, 1 point on line, 1229 other
  measures "d4" distance of L2.end L4.end
  measures "d5" distance from line of L6 L63.start
  measures "d8" distance of L63.start point (0, -32.85)
  measures "d15" distance of L15.start L64.end
  measures "d22" distance of L63.start L252.start
  measures "d29" distance of L357.end L491.start
extrude "Extrusion2" cut sketch "Sketch2" against normal blind 2
sketch "Sketch3" plane through (0, 0, 0) normal (0, -1, 0) x (1, 0, 0)
  line L0 (25.0493, 32.8498) -> (25.0493, -43.1502) projected
  line L1 (-23.9507, 32.8498) -> (25.0493, 32.8498) projected
  line L2 (-23.9507, -43.1502) -> (-23.9507, 32.8498) projected
  line L3 (25.0493, -43.1502) -> (-23.9507, -43.1502) projected
  line L4 (23.0493, -41.1502) -> (23.0493, 30.8498)
  line L5 (23.0493, 30.8498) -> (-21.9507, 30.8498)
  line L6 (-21.9507, 30.8498) -> (-21.9507, -41.1502)
  line L7 (-21.9507, -41.1502) -> (23.0493, -41.1502)
  point P0 (0, 0)
  dimension "d36" = 2
  constraints: 8 end point, 3 other
  measures "d36" distance between parallel lines of L0 L4
extrude "Extrusion3" add sketch "Sketch3" against normal blind 2
body "Solid1"
